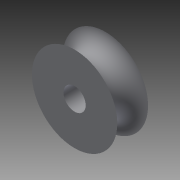
# Autodesk Inventor part: surgicalpulley
Saved by Autodesk Inventor 2015 (Build 190159000, 159)
## iProperties
Created: 2013-11-03
Part Number: surgicalpulley
Material: Generic
Document SubType Name: Modeling
Designer: jesse
Density: 1 g/cm^3
Appearance: Default
Author: jesse
Autodesk Inventor part; units mm, degrees
ref_plane "YZ Plane" through (0, 0, 0) normal (1, 0, 0) x (0, 1, 0)
ref_plane "XZ Plane" through (0, 0, 0) normal (0, 1, 0) x (-1, 0, 0)
ref_plane "XY Plane" through (0, 0, 0) normal (0, 0, 1) x (1, 0, 0)
sketch "Sketch1" plane through (0, 0, 0) normal (1, 0, 0) x (0, 1, 0)
  line L0 (-6.098, -7.32) -> (9.142, -7.32)
  line L1 (9.142, 5.08) -> (-6.098, 5.08)
  line L2 (9.142, 6.8113) -> (9.142, -7.738)
  arc A0 (-6.098, -7.32) -> (-6.098, 5.08) centre (-6.098, -1.12) ccw
  point P0 (0, 0)
  dimension "d4" = 12.4
  dimension "d5" = 15.24
  constraints: 6 end point, 3 point on circle, 2 point on line, 2 tangent, 1 centre point, 1 horizontal, 1 parallel
  measures "d4" distance between parallel lines of L0 L1
  measures "d5" distance of L1.start L1.end
revolve "Revolution1" add sketch "Sketch1" angle 360 about axis through (0, 9.142, 6.8113) along (0, 0, -1)
sketch "Sketch2" plane through (0, 9.142, -7.32) normal (0, 0, -1) x (-1, 0, 0)
  circle A0 centre (0, 0) radius 15.24 projected
  circle A1 centre (0, 0) radius 3.9688
  dimension "d1" = 7.9375
  constraints: 1 centre point, 1 coincident
  measures "d1" diameter of A1
extrude "Extrusion1" cut sketch "Sketch2" against normal through all contours A1
sketch "Sketch4" plane through (0, 0, 0) normal (1, 0, 0) x (0, 1, 0)
  line L0 (23.5043, 7.0392) -> (26.3008, 7.0392)
  line L1 (26.3008, 7.0392) -> (26.3008, -7.7625)
  line L2 (26.3008, -7.7625) -> (23.5043, -7.7625)
  line L3 (23.5043, -7.7625) -> (23.5043, 7.0392)
  line L4 (9.7561, -8.4) -> (9.7561, 8.96)
  point P0 (0, 0)
  constraints: 10 end point, 2 parallel, 1 horizontal, 1 perpendicular, 1 vertical, 2 other
revolve "Revolution2" cut sketch "Sketch4" angle 360 about axis through (0, 9.7561, -8.4) along (0, 0, 1)
body "Solid1"
